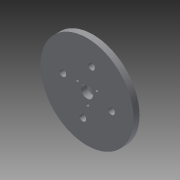
# Autodesk Inventor part: gearSpacerDisc01
Saved by Autodesk Inventor 2013 (Build 170138000, 138)
## iProperties
Created: 2014-07-01
Part Number: gearSpacerDisc01
Material: Generic
Document SubType Name: Modeling
Designer: Nano
Density: 1 g/cm^3
Author: Nano
Autodesk Inventor part; units mm, degrees
ref_plane "YZ Plane" through (0, 0, 0) normal (1, 0, 0) x (0, 1, 0)
ref_plane "XZ Plane" through (0, 0, 0) normal (0, 1, 0) x (-1, 0, 0)
ref_plane "XY Plane" through (0, 0, 0) normal (0, 0, 1) x (1, 0, 0)
ref_plane "Work Plane1" through (0, 0, 0) normal (0, 0, 1) x (1, 0, 0)
sketch "Sketch1" plane through (0, 0, 0) normal (0, 0, 1) x (1, 0, 0)
  circle A0 centre (0, 0) radius 3.175 projected
  circle A1 centre (0, 0) radius 24.765
  point P0 (0, 0)
  dimension "d0" = 49.53
  constraints: 1 centre point
  measures "d0" diameter of A1
extrude "Extrusion1" add sketch "Sketch1" along normal blind 3.175
sketch "Sketch2" plane through (0, 0, 0) normal (0, 0, -1) x (-1, 0, 0)
  circle A0 centre (12.9454, 2.2936) radius 1.8542
  circle A1 centre (-2.2936, 12.9454) radius 1.8542
  circle A2 centre (-12.9454, -2.2936) radius 1.8542
  circle A3 centre (2.2936, -12.9454) radius 1.8542
  constraints: 4 centre point, 8 other
extrude "Extrusion2" cut sketch "Sketch2" against normal through all
sketch "Sketch3" plane through (0, 0, 3.175) normal (0, 0, 1) x (1, 0, 0)
  circle A0 centre (-5.246, 2.7309) radius 0.762 projected
  circle A1 centre (4.988, 3.1777) radius 0.762 projected
  circle A2 centre (0.258, -5.9086) radius 0.762 projected
extrude "Extrusion3" cut sketch "Sketch3" against normal through all
body "Solid1"
